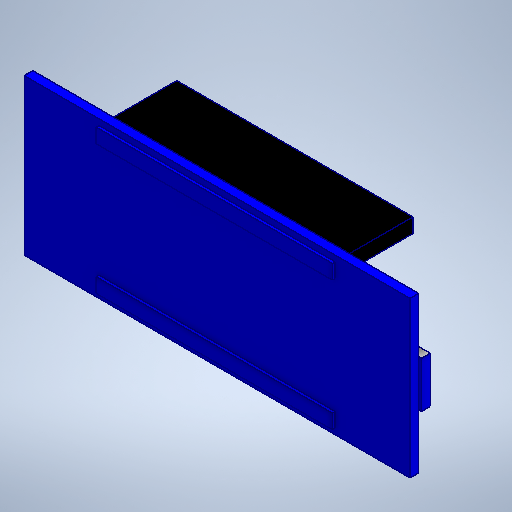
# Autodesk Inventor part: opencm9.04
Saved by Autodesk Inventor 2025 (Build 290162000, 162)
## iProperties
Created: 2025-10-18
Part Number: opencm9.04
Material: 一般
Document SubType Name: Modeling
Designer: sooo1
Density: 1 g/cm^3
Appearance: 既定
Author: sooo1
Autodesk Inventor part; units mm, degrees
ref_plane "YZ Plane" through (0, 0, 0) normal (1, 0, 0) x (0, 1, 0)
ref_plane "XZ Plane" through (0, 0, 0) normal (0, 1, 0) x (-1, 0, 0)
ref_plane "XY Plane" through (0, 0, 0) normal (0, 0, 1) x (1, 0, 0)
sketch "スケッチ1" plane through (0, 0, 0) normal (0, 0, 1) x (1, 0, 0)
  line L0 (-33.5, 13.5) -> (33.5, 13.5)
  line L1 (33.5, 13.5) -> (33.5, -13.5)
  line L2 (33.5, -13.5) -> (-33.5, -13.5)
  line L3 (-33.5, -13.5) -> (-33.5, 13.5)
  line L4 (-33.5, 13.5) -> (33.5, -13.5) construction
  line L5 (33.5, 13.5) -> (-33.5, -13.5) construction
  line L6 (-47, 0) -> (47.5, 0) construction
  line L7 (33.5, 4) -> (34, 4)
  line L8 (34, 4) -> (34, -4)
  line L9 (34, -4) -> (33.5, -4)
  line L10 (33.5, -4) -> (33.5, 4) construction
  line L11 (33.5, 4) -> (34, -4) construction
  line L12 (34, 4) -> (33.5, -4) construction
  line L13 (0, 18.9) -> (0, -18.9) construction
  line L14 (-20.5, 12.5) -> (20.5, 12.5)
  line L15 (20.5, 12.5) -> (20.5, 10)
  line L16 (20.5, 10) -> (-20.5, 10)
  line L17 (-20.5, 10) -> (-20.5, 12.5)
  line L18 (-20.5, 12.5) -> (20.5, 10) construction
  line L19 (20.5, 12.5) -> (-20.5, 10) construction
  line L20 (-20.5, -12.5) -> (20.5, -12.5)
  line L21 (20.5, -12.5) -> (20.5, -10)
  line L22 (20.5, -10) -> (-20.5, -10)
  line L23 (-20.5, -10) -> (-20.5, -12.5)
  line L24 (33.5, -4) -> (28.5, -4)
  line L25 (28.5, -4) -> (28.5, 4)
  line L26 (28.5, 4) -> (33.5, 4)
  point P0 (0, 0)
  point P1 (33.75, 0)
  point P2 (0, 11.25)
  dimension "d0" = 67
  dimension "d1" = 27
  dimension "d2" = 0.5
  dimension "d3" = 8
  dimension "d6" = 41
  dimension "d7" = 2.5
  dimension "d8" = 1
  dimension "d9" = 5
  constraints: 50 end point, 6 midpoint, 6 parallel, 5 perpendicular, 4 horizontal, 4 symmetric about line, 2 point on line, 1 collinear
  measures "d0" distance of L0.start L0.end
  measures "d1" distance of L2.end L0.start
  measures "d2" distance of L7.start L7.end
  measures "d3" distance of L7.end L8.end
  measures "d6" distance of L14.start L14.end
  measures "d7" distance of L16.end L14.start
  measures "d8" distance between parallel lines of L0 L14
  measures "d9" distance between parallel lines of L1 L25
extrude "押し出し1" add sketch "スケッチ1" along normal blind 1.5 contours L0 L1 L26 L25 L24 L2 L3 | L1 L24 L25 L26 | L14 L15 L16 L17 | L23 L22 L21 L20
extrude "押し出し2" add sketch "スケッチ1" against normal blind 1.5 contours L7 L8 L9 L1 | L1 L24 L25 L26
extrude "押し出し3" add sketch "スケッチ1" against normal blind 12 contours L14 L15 L16 L17 | L23 L22 L21 L20
extrude "押し出し4" add sketch "スケッチ1" along normal blind 2 contours L14 L15 L16 L17 | L23 L22 L21 L20
